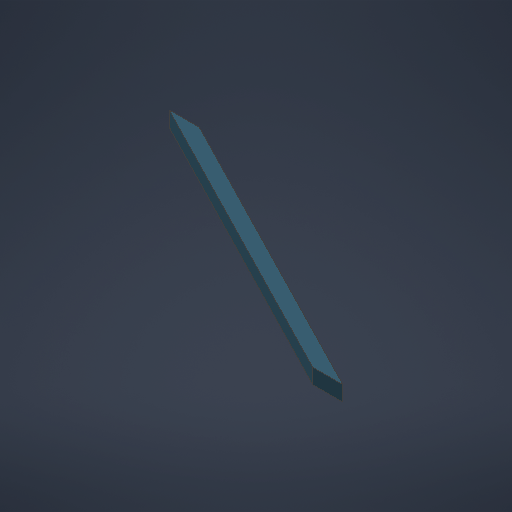
# Autodesk Inventor part: 2x4x(20x39)
Saved by Autodesk Inventor 2027 (Build 310192000, 192)
## iProperties
Created: 2026-05-29
Part Number: 2x4x(20x39)
Material: Generic
Document SubType Name: Modeling
Designer: lucas
Density: 1 g/cm^3
Appearance: Default
Author: lucas
Autodesk Inventor part; units mm, degrees
ref_plane "YZ Plane" through (0, 0, 0) normal (1, 0, 0) x (0, 1, 0)
ref_plane "XZ Plane" through (0, 0, 0) normal (0, 1, 0) x (-1, 0, 0)
ref_plane "XY Plane" through (0, 0, 0) normal (0, 0, 1) x (1, 0, 0)
sketch "Sketch1" plane through (0, 0, 0) normal (0, 1, 0) x (-1, 0, 0)
  line L0 (0, 0) -> (990.6, -508)
  line L1 (0, 0) -> (101.6, 0)
  line L2 (990.6, -508) -> (1092.2, -508)
  line L3 (101.6, 0) -> (1092.2, -508)
  point P0 (-50.7969, -505.4539)
  dimension "d0" = 508
  dimension "d1" = 1041.4
  dimension "d2" = 101.6
  dimension "d3" = 101.6
  constraints: 8 end point, 2 horizontal, 1 coincident
  measures "d0" distance of point (0, 0) point (-50.797, -505.454)
  measures "d1" distance of point (-50.797, -505.454) L0.end
  measures "d2" distance of L0.start L1.end
  measures "d3" distance of L0.end L2.end
extrude "Extrusion1" add sketch "Sketch1" along normal blind 50.8
body "Solid1"
